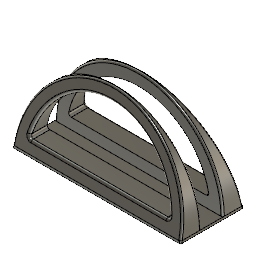
Dell Latitude E5470 Stand (Autodesk Fusion 360 design; units mm, degrees)
Autodesk Fusion 360 part; units mm, degrees
sketch "Sketch1" plane through (0, 0, 0) normal (0, 0, 1) x (1, 0, 0)
  line L0 (100, 37.5) -> (-100, 37.5)
  line L1 (-100, 37.5) -> (-100, -37.5)
  line L2 (-100, -37.5) -> (100, -37.5)
  line L3 (100, -37.5) -> (100, 37.5)
  line L4 (100, 37.5) -> (-100, -37.5) construction
  line L5 (-100, 37.5) -> (100, -37.5) construction
  dimension "d1" = 200
  dimension "d2" = 75
  constraint horizontal L0
  constraint perpendicular L0 L1
  constraint parallel L0 L2
  constraint parallel L1 L3
  constraint coincident L4 origin
  constraint coincident L5 origin
  measures "d1" distance of L1.end L2.end
  measures "d2" distance of L0.end L1.end
extrude "Extrude1" add sketch "Sketch1" along normal blind 3
sketch "Sketch2" plane through (0, 0, 3) normal (0, 0, 1) x (-1, 0, 0)
  line L0 (-100, 37.5) -> (-100, -37.5)
  line L1 (100, -37.5) -> (100, 37.5)
  line L2 (100, 37.5) -> (-100, 37.5)
  line L3 (-115, 12.775) -> (130, 12.775) construction
  line L4 (130, 12.775) -> (-100, 12.775)
  line L5 (-100, 12.775) -> (-100, 37.5)
  line L6 (-100, 37.5) -> (130, 37.5)
  line L7 (130, 37.5) -> (130, 12.775)
  line L8 (-20, 0) -> (-2.5, 0)
  line L9 (-100, -37.5) -> (130, -37.5)
  line L10 (-100, -12.775) -> (-100, -37.5)
  line L11 (130, -12.775) -> (-100, -12.775)
  line L12 (130, -37.5) -> (130, -12.775)
  dimension "d24" = 230
  dimension "d26" = 24.725
  constraint horizontal L3
  constraint horizontal L4
  constraint vertical L5
  constraint horizontal L6
  constraint vertical L7
  constraint coincident L0.start L2.end
  constraint symmetric L3.end L8 L11.start
  constraint symmetric L4.end L8 L10.start
  constraint symmetric L0.start L8 L0.end
  constraint symmetric L6.end L8 L9.end
  measures "d24" distance of L0.start L6.end
  measures "d26" distance of L3.end L6.end
extrude "Extrude2" add sketch "Sketch2" along normal blind 100 contours L0 L1 L2 L4 L5 L6 | L0 L1 L9 L10 L11
sketch "Sketch3" plane through (-100, 0, 0) normal (1, 0, 0) x (0, 1, 0)
  line L0 (37.5, 0) -> (-37.5, 0)
  line L1 (-37.5, 0) -> (-37.5, 103)
  line L2 (-12.775, 3) -> (12.775, 3)
  line L3 (12.775, 3) -> (12.775, 103)
  line L4 (-37.5, 103) -> (-12.775, 103)
  line L5 (37.5, 103) -> (37.5, 0)
  line L6 (16.8886, 103) -> (37.5, 3)
  line L7 (16.8886, 103) -> (37.5, 103)
  line L8 (37.5, 103) -> (37.5, 3)
  line L9 (0, 2.5) -> (0, 20)
  line L10 (-16.8886, 103) -> (-37.5, 103)
  line L11 (-37.5, 103) -> (-37.5, 3)
  line L12 (-16.8886, 103) -> (-37.5, 3)
  line L13 (12.775, 3) -> (37.5, 3) construction
  line L14 (-12.775, 103) -> (-12.775, 3)
  line L15 (12.775, 103) -> (37.5, 103)
  constraint coincident L5 L6.end
  constraint symmetric L5.start L9 L1.end
  constraint symmetric L9 L11.end L6.end
  constraint symmetric L6.start L9 L10.start
  constraint coincident L2.end L3.start
  constraint perpendicular L5 L13
extrude "Extrude5" cut sketch "Sketch3" along normal up to surface (200 mm away) contours L5 L6 L7 L8 L15 | L1 L4 L10 L11 L12
sketch "Sketch6" plane through (0, 12.775, 0) normal (0, -1, 0) x (1, 0, 0)
  line L0 (-100, 3) -> (100, 3)
  line L1 (100, 3) -> (100, 103)
  line L2 (100, 103) -> (-100, 103)
  line L3 (-100, 103) -> (-100, 3)
  line L4 (100, 3) -> (100, 103)
  line L5 (100, 103) -> (-100, 103)
  line L6 (-100, 103) -> (-100, 3)
  arc A0 (100, 3) -> (-100, 3) centre (0, 3) ccw
  arc A1 (84, 16) -> (-84, 16) centre (0, 3) ccw
  line L7 (-84, 16) -> (84, 16)
  constraint tangent L5 A0
  constraint coincident L0.end L1.start
  constraint coincident L0.start L3.end
  constraint concentric A0 A1
extrude "Extrude7" cut sketch "Sketch6" along normal up to surface and the other way up to surface contours L2 L3 L5 L6 A0 | L1 L2 L4 L5 A0 | A1 L7 end surface through (-100, -16.8886, 103) normal (0, -0.979412, 0.20187) offset 0 second end surface through (-100, 16.8886, 103) normal (0, 0.979412, 0.20187) offset 0
fillet "Fillet3" radius 2 4 edges at (0, -16.8886, 103) (0, -12.775, 103) (0, 12.775, 103) (0, 16.8886, 103)
fillet "Fillet3" radius 3 8 edges at (84, -23.7977, 16) (0, -19.9803, 88) (0, -34.8205, 16) (84, 23.7977, 16) (0, 34.8205, 16) (0, 19.9803, 88) (-84, -23.7977, 16) (-84, 23.7977, 16)
